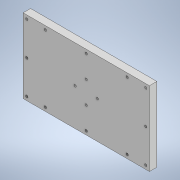
# Autodesk Inventor part: topwindow
Saved by Autodesk Inventor 2022.2 (Build 262287030, 287C)
## iProperties
Created: 2022-02-04
Part Number: topwindow
Material: Generic
Document SubType Name: Modeling
Designer: Tapendra
Density: 1 g/cm^3
Appearance: Default
Author: Tapendra
Autodesk Inventor part; units mm, degrees
ref_plane "YZ Plane" through (0, 0, 0) normal (1, 0, 0) x (0, 1, 0)
ref_plane "XZ Plane" through (0, 0, 0) normal (0, 1, 0) x (-1, 0, 0)
ref_plane "XY Plane" through (0, 0, 0) normal (0, 0, 1) x (1, 0, 0)
sketch "Sketch1" plane through (0, 0, 0) normal (0, 0, 1) x (1, 0, 0)
  line L0 (-85, 50) -> (85, 50)
  line L1 (85, 50) -> (85, -50)
  line L2 (85, -50) -> (-85, -50)
  line L3 (-85, -50) -> (-85, 50)
  line L4 (-85, 50) -> (85, -50) construction
  line L5 (85, 50) -> (-85, -50) construction
  point P0 (0, 0)
  dimension "d0" = 170
  dimension "d1" = 100
  constraints: 12 end point, 2 midpoint, 2 parallel, 1 horizontal, 1 perpendicular
  measures "d0" distance of L0.start L0.end
  measures "d1" distance of L0.end L1.end
extrude "Extrusion1" add sketch "Sketch1" along normal mid plane 10
sketch "Sketch2" plane through (0, 0, 5) normal (0, 0, 1) x (1, 0, 0)
  line L0 (-85, 50) -> (-85, -50) projected
  line L1 (-85, -50) -> (85, -50) projected
  line L2 (85, -50) -> (85, 50) projected
  line L3 (85, 50) -> (-85, 50) projected
  point P0 (0, 0)
  point P1 (-80, -45)
  point P2 (0, -45)
  point P3 (-55, -45)
  point P4 (55, -45)
  point P5 (0, -45)
  point P6 (80, -45)
  point P7 (-80, 0)
  point P8 (80, 0)
  point P9 (-80, 45)
  point P10 (80, 45)
  point P11 (-55, 45)
  point P12 (0, 45)
  point P13 (55, 45)
  dimension "d4" = 5
  dimension "d5" = 5
  dimension "d8" = 80
  dimension "d13" = 25
  dimension "d14" = 5
  dimension "d16" = 5
  dimension "d60" = 5
  dimension "d61" = 5
  dimension "d62" = 25
  dimension "d65" = 45
  dimension "d72" = 90
  constraints: 2 vertical, 1 coincident, 7 other
  measures "d4" distance from line of point (-80, -45) L0
  measures "d5" distance from line of L1 point (-80, -45)
  measures "d8" distance of point (-80, -45) point (0, -45)
  measures "d13" distance of point (-80, -45) point (-55, -45)
  measures "d14" distance from line of L1 point (-55, -45)
  measures "d16" distance from line of L1 point (55, -45)
  measures "d60" distance from line of point (80, -45) L2
  measures "d61" distance from line of point (80, -45) L1
  measures "d62" distance of point (55, -45) point (80, -45)
  measures "d65" distance of point (-80, -45) point (-80, 0)
  measures "d72" distance of point (-55, -45) point (-55, 45)
hole "Hole1" at (-80, -45, 5) at (0, -45, 5) at (-55, -45, 5) at (55, -45, 5) at (-80, 45, 5) at (-80, 0, 5) at (-55, 45, 5) at (0, 45, 5) at (55, 45, 5) at (80, 45, 5) at (80, 0, 5) at (80, -45, 5) direction (0, 0, -1) diameter 3.242 end through all thread size "M4x0.7" class "6H" standard "ANSI Metric M Profile"
sketch "Sketch3" plane through (0, 0, 5) normal (0, 0, 1) x (1, 0, 0)
  point P0 (0, 0)
  point P1 (0, 15)
  point P2 (-15, 0)
  point P3 (0, -15)
  point P4 (15, 0)
  dimension "d105" = 15
  dimension "d108" = 360
  constraints: 1 vertical alignment, 5 other
  measures "d105" distance of point (0, 15) point (0, 0)
hole "Hole2" at (0, 15, 5) at (-15, 0, 5) at (0, -15, 5) at (15, 0, 5) direction (0, 0, -1) diameter 3 depth 5 tip angle 118
body "Solid1"
